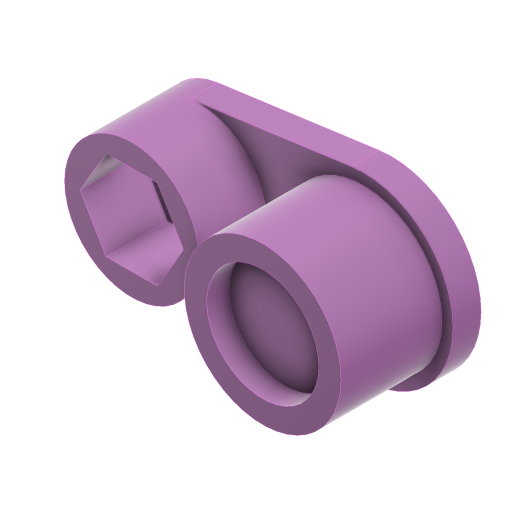
# Autodesk Inventor part: Капсуль
Saved by Autodesk Inventor 2023 (Build 270158000, 158)
## iProperties
Created: 2023-03-23
Part Number: Капсуль
Material: Типовые
Document SubType Name: Modeling
Designer: Admin
Density: 1 g/cm^3
Appearance: По умолчанию
Author: Admin
Autodesk Inventor part; units mm, degrees
ref_plane "YZ Plane" through (0, 0, 0) normal (1, 0, 0) x (0, 1, 0)
ref_plane "XZ Plane" through (0, 0, 0) normal (0, 1, 0) x (-1, 0, 0)
ref_plane "XY Plane" through (0, 0, 0) normal (0, 0, 1) x (1, 0, 0)
sketch "Эскиз1" plane through (0, 0, 0) normal (0, 0, 1) x (1, 0, 0)
  circle A0 centre (0, 0) radius 7
  circle A1 centre (0, 0) radius 8
  circle A2 centre (-14.6897, 0) radius 2.5
  circle A3 centre (-14.6897, 0) radius 6
  line L0 (-18.6897, -2.3094) -> (-18.6897, 2.3094)
  line L1 (-18.6897, 2.3094) -> (-14.6897, 4.6188)
  line L2 (-14.6897, 4.6188) -> (-10.6897, 2.3094)
  line L3 (-10.6897, 2.3094) -> (-10.6897, -2.3094)
  line L4 (-10.6897, -2.3094) -> (-14.6897, -4.6188)
  line L5 (-14.6897, -4.6188) -> (-18.6897, -2.3094)
  line L6 (-1.0892, -7.9255) -> (-15.5066, -5.9441)
  line L7 (-1.0892, 7.9255) -> (-15.5066, 5.9441)
  circle A4 centre (0, 0) radius 5
  dimension "d10" = 5
  dimension "d11" = 2
  dimension "d14" = 14.6897
  dimension "Magnet_fit" = 10
  constraints: 16 end point, 5 centre point, 5 coincident, 4 point on circle, 4 tangent, 1 horizontal alignment, 1 parallel, 1 vertical, 15 other
  measures "d10" diameter of A2
  measures "d11" distance edge to line of A3 L1
  measures "d14" distance of point (-14.69, 0) A0.centre
  measures "Magnet_fit" diameter of A4
extrude "Выдавливание1" add sketch "Эскиз1" against normal blind 2.5 contours A0 | A1 | A1 L6 A3 L7 | A3 | A2 | L0 L1 L2 L3 L4 L5 | A4
extrude "Выдавливание2" cut sketch "Эскиз1" against normal blind 1 contours A2
extrude "Выдавливание3" add sketch "Эскиз1" along normal blind 0.5 contours A3 | L0 L1 L2 L3 L4 L5
sketch "Эскиз2" plane through (-14.6897, 0, 0.5) normal (0, 0, 1) x (1, 0, 0)
  line L0 (-2.3094, 4) -> (2.3094, 4)
  line L1 (2.3094, 4) -> (4.6188, 0)
  line L2 (4.6188, 0) -> (2.3094, -4)
  line L3 (2.3094, -4) -> (-2.3094, -4)
  line L4 (-2.3094, -4) -> (-4.6188, 0)
  line L5 (-4.6188, 0) -> (-2.3094, 4)
  circle A0 centre (0, 0) radius 6 projected
  point P0 (14.6897, 0)
  point P1 (0, 0)
  dimension "d21" = 8
  constraints: 12 end point, 1 coincident, 1 horizontal, 13 other
  measures "d21" distance between parallel lines of L1 L4
extrude "Выдавливание4" add sketch "Эскиз2" along normal blind 5.5
extrude "Выдавливание5" add sketch "Эскиз1" along normal blind 9 contours A0
extrude "Выдавливание6" add sketch "Эскиз1" along normal blind 7 contours A4
